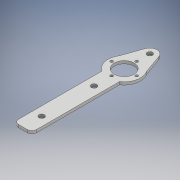
# Autodesk Inventor part: spinnyBoiPlate
Saved by Autodesk Inventor 2018.3 (Build 223284000, 284)
## iProperties
Created: 2018-08-05
Part Number: spinnyBoiPlate
Material: Generic
Document SubType Name: Modeling
Designer: mzhang
Density: 1 g/cm^3
Appearance: Default
Author: mzhang
Autodesk Inventor part; units mm, degrees
ref_plane "YZ Plane" through (0, 0, 0) normal (1, 0, 0) x (0, 1, 0)
ref_plane "XZ Plane" through (0, 0, 0) normal (0, 1, 0) x (-1, 0, 0)
ref_plane "XY Plane" through (0, 0, 0) normal (0, 0, 1) x (1, 0, 0)
sketch "Sketch2" plane through (0, 0, 0) normal (0, 0, 1) x (1, 0, 0)
  circle A0 centre (0, 0) radius 3
  circle A1 centre (0, 58.42) radius 3
  line L0 (0, 58.42) -> (0, 0)
  line L1 (9.9209, -20.79) -> (-10, -20.79)
  line L2 (-10, -20.79) -> (-10, 77.0383)
  line L3 (9.9209, 76.9858) -> (9.9209, -20.79)
  circle A2 centre (0, 92) radius 11.049
  circle A3 centre (0, 105.9954) radius 1.55
  circle A4 centre (-13.9954, 92) radius 1.55
  circle A5 centre (0, 78.0046) radius 1.55
  circle A6 centre (13.9954, 92) radius 1.55
  circle A7 centre (0, 120.5812) radius 3
  arc A8 (9.9209, 76.9858) -> (15.1304, 101.7428) centre (0, 92) ccw
  arc A9 (-15.1304, 101.7428) -> (-10, 77.0383) centre (0, 92) ccw
  arc A10 (7.5442, 123.2432) -> (-7.5442, 123.2432) centre (0, 120.5812) ccw
  line L4 (-15.1304, 101.7428) -> (-7.5442, 123.2432)
  line L5 (15.1304, 101.7428) -> (7.5442, 123.2432)
  point P0 (0, 29.21)
  dimension "d47" = 6
  dimension "d51" = 6
  dimension "d56" = 22.098
  dimension "d58" = 3.1
  dimension "d61" = 360
  dimension "d63" = 6
  dimension "d64" = 13.9954
  dimension "d65" = 5
  constraints: 12 end point, 11 centre point, 6 point on circle, 2 coincident, 2 tangent, 1 horizontal, 1 midpoint, 1 parallel, 1 perpendicular, 1 vertical, 9 other
  measures "d47" diameter of A0
  measures "d51" diameter of A1
  measures "d56" diameter of A2
  measures "d58" diameter of A3
  measures "d63" diameter of A7
  measures "d64" horizontal distance of A6.centre A7.centre
  measures "d65" radial gap between concentric circles of A7 A10
extrude "Extrusion2" add sketch "Sketch2" along normal blind 3.175
fillet "Fillet1" radius 5 2 edges at (9.9209, -20.79, 1.5875) (-10, -20.79, 1.5875)
body "Solid2"
